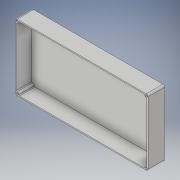
# Autodesk Inventor part: electronics_box
Saved by Autodesk Inventor 2019.4 (Build 234330000, 330)
## iProperties
Created: 2020-10-01
Part Number: electronics_box
Material: Generic
Document SubType Name: Modeling
Designer: deanv
Density: 1 g/cm^3
Appearance: Default
Author: deanv
Autodesk Inventor part; units mm, degrees
ref_plane "YZ Plane" through (0, 0, 0) normal (1, 0, 0) x (0, 1, 0)
ref_plane "XZ Plane" through (0, 0, 0) normal (0, 1, 0) x (-1, 0, 0)
ref_plane "XY Plane" through (0, 0, 0) normal (0, 0, 1) x (1, 0, 0)
sketch "Sketch1" plane through (0, 0, 0) normal (0, 0, 1) x (1, 0, 0)
  line L0 (-150, -75) -> (150, -75) construction
  line L1 (150, -75) -> (150, 75) construction
  line L2 (150, 75) -> (-150, 75) construction
  line L3 (-150, 75) -> (-150, -75) construction
  line L4 (-150, -75) -> (150, 75) construction
  line L5 (150, -75) -> (-150, 75) construction
  line L6 (147.5, -72.5) -> (-147.5, -72.5) construction
  line L7 (-147.5, -72.5) -> (-147.5, 72.5) construction
  line L8 (-147.5, 72.5) -> (147.5, 72.5) construction
  line L9 (147.5, 72.5) -> (147.5, -72.5) construction
  line L10 (147.5, -72.5) -> (-147.5, 72.5) construction
  line L11 (-147.5, -72.5) -> (147.5, 72.5) construction
  line L12 (-150, 75) -> (-146, 75) construction
  line L13 (-146, 75) -> (-146, 71) construction
  line L14 (-146, 71) -> (-150, 71) construction
  line L15 (-150, 71) -> (-150, 75) construction
  arc A0 (-146, 75) -> (-150, 71) centre (-146, 71) ccw
  line L16 (-150, -75) -> (-146, -75) construction
  line L17 (-146, -75) -> (-146, -71) construction
  line L18 (-146, -71) -> (-150, -71) construction
  line L19 (-150, -71) -> (-150, -75) construction
  line L20 (150, -75) -> (146, -75) construction
  line L21 (146, -75) -> (146, -71) construction
  line L22 (146, -71) -> (150, -71) construction
  line L23 (150, -71) -> (150, -75) construction
  line L24 (150, 75) -> (146, 75) construction
  line L25 (146, 75) -> (146, 71) construction
  line L26 (146, 71) -> (150, 71) construction
  line L27 (150, 71) -> (150, 75) construction
  line L28 (-146, 75) -> (146, 75)
  arc A1 (150, 71) -> (146, 75) centre (146, 71) ccw
  line L29 (150, 71) -> (150, -71)
  arc A2 (146, -75) -> (150, -71) centre (146, -71) ccw
  line L30 (146, -75) -> (-146, -75)
  arc A3 (-150, -71) -> (-146, -75) centre (-146, -71) ccw
  line L31 (-150, -71) -> (-150, 71)
  circle A4 centre (-146, 71) radius 2.5
  circle A5 centre (-146, -71) radius 2.5
  circle A6 centre (146, -71) radius 2.5
  circle A7 centre (146, 71) radius 2.5
  line L32 (-146, 71) -> (-142, 71) construction
  line L33 (-142, 71) -> (-142, 67) construction
  line L34 (-142, 67) -> (-146, 67) construction
  line L35 (-146, 67) -> (-146, 71) construction
  line L36 (-146, -71) -> (-142, -71) construction
  line L37 (-142, -71) -> (-142, -67) construction
  line L38 (-142, -67) -> (-146, -67) construction
  line L39 (-146, -67) -> (-146, -71) construction
  line L40 (146, -71) -> (142, -71) construction
  line L41 (142, -71) -> (142, -67) construction
  line L42 (142, -67) -> (146, -67) construction
  line L43 (146, -67) -> (146, -71) construction
  line L44 (146, 71) -> (142, 71) construction
  line L45 (142, 71) -> (142, 67) construction
  line L46 (142, 67) -> (146, 67) construction
  line L47 (146, 67) -> (146, 71) construction
  arc A8 (-146, 67) -> (-142, 71) centre (-146, 71) ccw
  arc A9 (-142, -71) -> (-146, -67) centre (-146, -71) ccw
  arc A10 (146, -67) -> (142, -71) centre (146, -71) ccw
  arc A11 (142, 71) -> (146, 67) centre (146, 71) ccw
  line L48 (-142, 71) -> (-140.5, 71) construction
  line L49 (-140.5, 71) -> (-140.5, 72.5) construction
  line L50 (-140.5, 72.5) -> (-142, 72.5) construction
  line L51 (-142, 72.5) -> (-142, 71) construction
  line L52 (-146, 67) -> (-147.5, 67) construction
  line L53 (-147.5, 67) -> (-147.5, 65.5) construction
  line L54 (-147.5, 65.5) -> (-146, 65.5) construction
  line L55 (-146, 65.5) -> (-146, 67) construction
  line L56 (142, 71) -> (140.5, 71) construction
  line L57 (140.5, 71) -> (140.5, 72.5) construction
  line L58 (140.5, 72.5) -> (142, 72.5) construction
  line L59 (142, 72.5) -> (142, 71) construction
  line L60 (146, 67) -> (147.5, 67) construction
  line L61 (147.5, 67) -> (147.5, 65.5) construction
  line L62 (147.5, 65.5) -> (146, 65.5) construction
  line L63 (146, 65.5) -> (146, 67) construction
  line L64 (146, -67) -> (147.5, -67) construction
  line L65 (147.5, -67) -> (147.5, -65.5) construction
  line L66 (147.5, -65.5) -> (146, -65.5) construction
  line L67 (146, -65.5) -> (146, -67) construction
  line L68 (142, -71) -> (140.5, -71) construction
  line L69 (140.5, -71) -> (140.5, -72.5) construction
  line L70 (140.5, -72.5) -> (142, -72.5) construction
  line L71 (142, -72.5) -> (142, -71) construction
  line L72 (-142, -71) -> (-140.5, -71) construction
  line L73 (-140.5, -71) -> (-140.5, -72.5) construction
  line L74 (-140.5, -72.5) -> (-142, -72.5) construction
  line L75 (-142, -72.5) -> (-142, -71) construction
  line L76 (-146, -67) -> (-147.5, -67) construction
  line L77 (-147.5, -67) -> (-147.5, -65.5) construction
  line L78 (-147.5, -65.5) -> (-146, -65.5) construction
  line L79 (-146, -65.5) -> (-146, -67) construction
  arc A12 (-147.5, -65.5) -> (-146, -67) centre (-146, -65.5) ccw
  arc A13 (-142, -71) -> (-140.5, -72.5) centre (-140.5, -71) ccw
  arc A14 (-140.5, 72.5) -> (-142, 71) centre (-140.5, 71) ccw
  arc A15 (-146, 67) -> (-147.5, 65.5) centre (-146, 65.5) ccw
  arc A16 (140.5, -72.5) -> (142, -71) centre (140.5, -71) ccw
  arc A17 (146, -67) -> (147.5, -65.5) centre (146, -65.5) ccw
  line L80 (147.5, -65.5) -> (147.5, 65.5)
  arc A18 (147.5, 65.5) -> (146, 67) centre (146, 65.5) ccw
  arc A19 (142, 71) -> (140.5, 72.5) centre (140.5, 71) ccw
  line L81 (140.5, 72.5) -> (-140.5, 72.5)
  line L82 (-147.5, 65.5) -> (-147.5, -65.5)
  line L83 (-140.5, -72.5) -> (140.5, -72.5)
  line L84 (146, 75) -> (-146, 75)
  arc A20 (-146, 75) -> (-150, 71) centre (-146, 71) ccw
  line L85 (-150, 71) -> (-150, -71)
  arc A21 (-150, -71) -> (-146, -75) centre (-146, -71) ccw
  line L86 (-146, -75) -> (146, -75)
  arc A22 (146, -75) -> (150, -71) centre (146, -71) ccw
  line L87 (150, -71) -> (150, 71)
  arc A23 (150, 71) -> (146, 75) centre (146, 71) ccw
  arc A24 (142, 71) -> (146, 67) centre (146, 71) ccw
  arc A25 (142, 71) -> (140.5, 72.5) centre (140.5, 71) ccw
  line L88 (140.5, 72.5) -> (-140.5, 72.5)
  arc A26 (-140.5, 72.5) -> (-142, 71) centre (-140.5, 71) ccw
  arc A27 (-146, 67) -> (-142, 71) centre (-146, 71) ccw
  arc A28 (-146, 67) -> (-147.5, 65.5) centre (-146, 65.5) ccw
  line L89 (-147.5, 65.5) -> (-147.5, -65.5)
  arc A29 (-147.5, -65.5) -> (-146, -67) centre (-146, -65.5) ccw
  arc A30 (-142, -71) -> (-146, -67) centre (-146, -71) ccw
  arc A31 (-142, -71) -> (-140.5, -72.5) centre (-140.5, -71) ccw
  line L90 (-140.5, -72.5) -> (140.5, -72.5)
  arc A32 (140.5, -72.5) -> (142, -71) centre (140.5, -71) ccw
  arc A33 (146, -67) -> (142, -71) centre (146, -71) ccw
  arc A34 (146, -67) -> (147.5, -65.5) centre (146, -65.5) ccw
  line L91 (147.5, -65.5) -> (147.5, 65.5)
  arc A35 (147.5, 65.5) -> (146, 67) centre (146, 65.5) ccw
  point P0 (0, 0)
  dimension "d0" = 300
  dimension "d1" = 150
  dimension "d2" = 295
  dimension "d3" = 145
  dimension "d4" = 4
  dimension "d5" = 4
  dimension "d6" = 4
  dimension "d7" = 4
  dimension "d8" = 4
  dimension "d9" = 4
  dimension "d10" = 4
  dimension "d11" = 4
  dimension "d12" = 4
  dimension "d13" = 4
  dimension "d14" = 4
  dimension "d15" = 4
  dimension "d16" = 5
  dimension "d17" = 5
  dimension "d18" = 5
  dimension "d19" = 5
  dimension "d20" = 4
  dimension "d21" = 4
  dimension "d22" = 4
  dimension "d23" = 4
  dimension "d24" = 4
  dimension "d25" = 4
  dimension "d26" = 4
  dimension "d27" = 4
  dimension "d28" = 4
  dimension "d29" = 4
  dimension "d30" = 4
  dimension "d31" = 4
  dimension "d32" = 1.5
  dimension "d33" = 1.5
  dimension "d34" = 1.5
  dimension "d35" = 1.5
  dimension "d36" = 1.5
  dimension "d37" = 1.5
  dimension "d38" = 1.5
  dimension "d39" = 1.5
  dimension "d40" = 1.5
  dimension "d41" = 1.5
  dimension "d42" = 1.5
  dimension "d43" = 1.5
  dimension "d44" = 1.5
  dimension "d45" = 1.5
  dimension "d46" = 1.5
  dimension "d47" = 1.5
  dimension "d48" = 1.5
  dimension "d49" = 1.5
  dimension "d50" = 1.5
  dimension "d51" = 1.5
  dimension "d52" = 1.5
  dimension "d53" = 1.5
  dimension "d54" = 1.5
  dimension "d55" = 1.5
  constraints: 184 end point, 64 point on circle, 36 centre point, 36 parallel, 19 horizontal, 19 perpendicular, 9 tangent, 8 collinear, 7 concentric, 5 point on line, 4 coincident, 4 midpoint
  measures "d0" distance of L2.end L1.end
  measures "d1" distance of L1.end L0.end
  measures "d2" distance of L7.end L8.end
  measures "d3" distance between parallel lines of L6 L8
  measures "d4" distance of L13.end L14.end
  measures "d5" distance of L12.end L13.end
  measures "d6" radius of A0
  measures "d7" distance of L18.end L17.end
  measures "d8" distance of L17.end L16.end
  measures "d9" distance of L21.end L22.end
  measures "d10" distance of L20.end L21.end
  measures "d11" distance of L26.end L25.end
  measures "d12" distance of L25.end L24.end
  measures "d13" radius of A1
  measures "d14" radius of A2
  measures "d15" radius of A3
  measures "d16" diameter of A4
  measures "d17" diameter of A5
  measures "d18" diameter of A6
  measures "d19" diameter of A7
  measures "d20" distance of L33.end L34.end
  measures "d21" distance of L32.end L33.end
  measures "d22" distance of L38.end L37.end
  measures "d23" distance of L37.end L36.end
  measures "d24" distance of L41.end L42.end
  measures "d25" distance of L40.end L41.end
  measures "d26" distance of L46.end L45.end
  measures "d27" distance of L45.end L44.end
  measures "d28" radius of A8
  measures "d29" radius of A9
  measures "d30" radius of A10
  measures "d31" radius of A11
  measures "d32" distance of L50.end L49.end
  measures "d33" distance of L49.end L48.end
  measures "d34" distance of L54.end L53.end
  measures "d35" distance of L53.end L52.end
  measures "d36" distance of L57.end L58.end
  measures "d37" distance of L56.end L57.end
  measures "d38" distance of L61.end L62.end
  measures "d39" distance of L60.end L61.end
  measures "d40" distance of L66.end L65.end
  measures "d41" distance of L65.end L64.end
  measures "d42" distance of L70.end L69.end
  measures "d43" distance of L69.end L68.end
  measures "d44" distance of L73.end L74.end
  measures "d45" distance of L72.end L73.end
  measures "d46" distance of L77.end L78.end
  measures "d47" distance of L76.end L77.end
  measures "d48" radius of A12
  measures "d49" radius of A13
  measures "d50" radius of A14
  measures "d51" radius of A15
  measures "d52" radius of A16
  measures "d53" radius of A17
  measures "d54" radius of A18
  measures "d55" radius of A19
extrude "Extrusion1" add sketch "Sketch1" along normal blind 2.5 contours L28 A1 L29 A2 L30 A3 L31 A0 | A8 A14 L81 A19 A11 A18 L80 A17 A10 A16 L83 A13 A9 A12 L82 A15
extrude "Extrusion2" add sketch "Sketch1" along normal blind 37.5
extrude "Extrusion3" add sketch "Sketch1" along normal blind 35.5 contours A4 | A5 | A6 | A7
equation "\"d21\" = d20"
body "Solid1"
